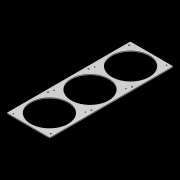
# Autodesk Inventor part: front_140mm
Saved by Autodesk Inventor 2018 (Build 220112000, 112)
## iProperties
Created: 2020-10-17
Part Number: front_140mm
Material: アルミニウム 6061
Document SubType Name: Modeling
Designer: gisen
Density: 2.7 g/cm^3
Appearance: アルミニウム - フラット
Author: gisen
Autodesk Inventor part; units mm, degrees
ref_plane "YZ Plane" through (0, 0, 0) normal (1, 0, 0) x (0, 1, 0)
ref_plane "XZ Plane" through (0, 0, 0) normal (0, 1, 0) x (-1, 0, 0)
ref_plane "XY Plane" through (0, 0, 0) normal (0, 0, 1) x (1, 0, 0)
sketch "スケッチ1" plane through (0, 0, 0) normal (0, 0, 1) x (1, 0, 0)
  line L0 (-75, -215) -> (75, -215)
  line L1 (75, -215) -> (75, 215)
  line L2 (75, 215) -> (-75, 215)
  line L3 (-75, 215) -> (-75, -215)
  line L4 (-75, -215) -> (75, 215) construction
  line L5 (75, -215) -> (-75, 215) construction
  line L6 (-65, -215) -> (-65, 215) construction
  line L7 (-65, 59.8957) -> (59.8957, 65) construction
  line L8 (59.8957, 65) -> (65, -59.8957) construction
  line L9 (65, -59.8957) -> (-59.8957, -65) construction
  line L10 (-59.8957, -65) -> (-65, 59.8957) construction
  line L11 (-65, 59.8957) -> (65, -59.8957) construction
  line L12 (59.8957, 65) -> (-59.8957, -65) construction
  circle A0 centre (-65, 59.8957) radius 2.25
  line L13 (-67.0832, -72.8) -> (72.8, -67.0832) construction
  line L14 (72.8, -67.0832) -> (67.0832, 72.8) construction
  line L15 (67.0832, 72.8) -> (-72.8, 67.0832) construction
  line L16 (-72.8, 67.0832) -> (-67.0832, -72.8) construction
  line L17 (-67.0832, -72.8) -> (67.0832, 72.8) construction
  line L18 (72.8, -67.0832) -> (-72.8, 67.0832) construction
  line L19 (0, 0) -> (0, 70.0584) construction
  circle A1 centre (65, -59.8957) radius 2.25
  circle A2 centre (59.8957, 65) radius 1.6
  circle A3 centre (-59.8957, -65) radius 1.6
  circle A4 centre (0, 0) radius 65
  circle A5 centre (59.8957, 206) radius 1.6
  circle A6 centre (0, 141) radius 65
  circle A7 centre (-65, 200.8957) radius 2.25
  circle A8 centre (-59.8957, 76) radius 1.6
  circle A9 centre (65, 81.1043) radius 2.25
  line L20 (0, 141) -> (0, 211.0584) construction
  circle A10 centre (59.8957, -76) radius 1.6
  circle A11 centre (0, -141) radius 65
  circle A12 centre (-65, -81.1043) radius 2.25
  circle A13 centre (-59.8957, -206) radius 1.6
  circle A14 centre (65, -200.8957) radius 2.25
  line L21 (0, -141) -> (0, -70.9416) construction
  circle A15 centre (59.8957, 65) radius 1.6
  circle A16 centre (0, 0) radius 65
  circle A17 centre (-65, 59.8957) radius 2.25
  circle A18 centre (-59.8957, -65) radius 1.6
  circle A19 centre (65, -59.8957) radius 2.25
  line L22 (0, 0) -> (0, 70.0584) construction
  dimension "d0" = 150
  dimension "d1" = 430
  dimension "d3" = 65
  dimension "d4" = 125
  dimension "d7" = 4.5
  dimension "d8" = 140
  dimension "d9" = 70.0584
  dimension "d10" = 3.2
  dimension "d11" = 130
  dimension "d14" = 141
  dimension "d17" = 141
  constraints: 46 end point, 20 centre point, 8 coincident, 7 parallel, 6 midpoint, 6 perpendicular, 4 point on line, 3 vertical, 2 collinear, 2 equal radius, 1 horizontal, 37 other
  measures "d0" distance of L2.end L1.end
  measures "d1" distance of L1.end L0.end
  measures "d3" distance from line of L19.start L6
  measures "d4" distance of L7.end L8.end
  measures "d7" diameter of A0
  measures "d8" distance of L14.end L13.end
  measures "d9" distance of L19.start L19.end
  measures "d10" diameter of A2
  measures "d11" diameter of A4
  measures "d14" distance of A2.centre A5.centre
  measures "d17" distance of A2.centre A10.centre
extrude "押し出し1" add sketch "スケッチ1" along normal blind 3
fillet "フィレット1" radius 3 4 edges at (-75, 215, 1.5) (75, 215, 1.5) (-75, -215, 1.5) (75, -215, 1.5)
